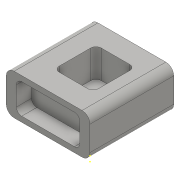
# Autodesk Inventor part: PassengerSection
Saved by Autodesk Inventor 2016 (Build 200138000, 138)
## iProperties
Created: 2016-01-08
Part Number: PassengerSection
Material: Generic
Document SubType Name: Modeling
Designer: 301278
Density: 1 g/cm^3
Appearance: Default
Author: 301278
Autodesk Inventor part; units mm, degrees
ref_plane "YZ Plane" through (0, 0, 0) normal (1, 0, 0) x (0, 1, 0)
ref_plane "XZ Plane" through (0, 0, 0) normal (0, 1, 0) x (-1, 0, 0)
ref_plane "XY Plane" through (0, 0, 0) normal (0, 0, 1) x (1, 0, 0)
sketch "Sketch1" plane through (0, 0, 0) normal (0, 0, 1) x (1, 0, 0)
  point P0 (0, 0)
sketch "Sketch2" plane through (0, 0, 0) normal (0, 0, 1) x (1, 0, 0)
  line L0 (7.62, 0) -> (72.898, 0)
  line L1 (80.518, 7.62) -> (80.518, 31.242)
  line L2 (72.898, 38.862) -> (7.62, 38.862)
  line L3 (0, 31.242) -> (0, 7.62)
  arc A0 (7.62, 38.862) -> (0, 31.242) centre (7.62, 31.242) ccw
  arc A1 (80.518, 31.242) -> (72.898, 38.862) centre (72.898, 31.242) ccw
  arc A2 (72.898, 0) -> (80.518, 7.62) centre (72.898, 7.62) ccw
  arc A3 (0, 7.62) -> (7.62, 0) centre (7.62, 7.62) ccw
  point P0 (0, 0)
  point P1 (80.518, 38.862)
  point P2 (80.518, 0)
  point P3 (0, 38.862)
  dimension "d0" = 80.518
  dimension "d1" = 38.862
  dimension "d2" = 7.62
  dimension "d3" = 7.62
  constraints: 8 end point, 8 point on circle, 8 point on line, 8 tangent, 4 centre point, 2 equal radius, 2 parallel, 1 horizontal, 1 perpendicular
  measures "d0" distance of point (0, 38.862) point (80.518, 38.862)
  measures "d1" distance of point (80.518, 38.862) point (80.518, 0)
  measures "d2" radius of A0
  measures "d3" radius of A1
extrude "Extrusion1" add sketch "Sketch2" along normal blind 80.518
sketch "Sketch3" plane through (0, 0, 80.518) normal (0, 0, 1) x (1, 0, 0)
  line L0 (13.716, 32.004) -> (66.802, 32.004)
  line L1 (71.882, 26.924) -> (71.882, 10.16)
  line L2 (66.802, 5.08) -> (13.716, 5.08)
  line L3 (8.636, 10.16) -> (8.636, 26.924)
  arc A0 (13.716, 32.004) -> (8.636, 26.924) centre (13.716, 26.924) ccw
  arc A1 (71.882, 26.924) -> (66.802, 32.004) centre (66.802, 26.924) ccw
  arc A2 (66.802, 5.08) -> (71.882, 10.16) centre (66.802, 10.16) ccw
  arc A3 (8.636, 10.16) -> (13.716, 5.08) centre (13.716, 10.16) ccw
  line L4 (72.898, 38.862) -> (7.62, 38.862) projected
  line L5 (0, 31.242) -> (0, 7.62) projected
  line L6 (80.518, 7.62) -> (80.518, 31.242) projected
  line L7 (72.898, 0) -> (7.62, 0) projected
  point P0 (0, 0)
  dimension "d6" = 5.08
  dimension "d7" = 5.08
  dimension "d8" = 6.858
  dimension "d9" = 8.636
  dimension "d10" = 8.636
  dimension "d11" = 5.08
  constraints: 8 end point, 8 point on circle, 8 tangent, 4 centre point, 2 equal radius, 2 parallel, 1 horizontal, 1 perpendicular
  measures "d6" radius of A0
  measures "d7" radius of A1
  measures "d8" distance between parallel lines of L4 L0
  measures "d9" distance between parallel lines of L5 L3
  measures "d10" distance between parallel lines of L6 L1
  measures "d11" distance from line of L7 L2.start
extrude "Extrusion2" cut sketch "Sketch3" against normal blind 14.478
sketch "Sketch4" plane through (0, 0, 0) normal (0, 0, -1) x (-1, 0, 0)
  line L0 (-65.659, 33.782) -> (-14.859, 33.782)
  line L1 (-9.779, 28.702) -> (-9.779, 10.16)
  line L2 (-14.859, 5.08) -> (-65.659, 5.08)
  line L3 (-70.739, 10.16) -> (-70.739, 28.702)
  arc A0 (-65.659, 33.782) -> (-70.739, 28.702) centre (-65.659, 28.702) ccw
  arc A1 (-70.739, 10.16) -> (-65.659, 5.08) centre (-65.659, 10.16) ccw
  arc A2 (-14.859, 5.08) -> (-9.779, 10.16) centre (-14.859, 10.16) ccw
  arc A3 (-9.779, 28.702) -> (-14.859, 33.782) centre (-14.859, 28.702) ccw
  line L4 (-7.62, 38.862) -> (-72.898, 38.862) projected
  line L5 (-72.898, 0) -> (-7.62, 0) projected
  line L6 (0, 7.62) -> (0, 31.242) projected
  line L7 (-80.518, 31.242) -> (-80.518, 7.62) projected
  point P0 (0, 0)
  dimension "d14" = 5.08
  dimension "d15" = 5.08
  dimension "d16" = 5.08
  dimension "d17" = 9.779
  dimension "d18" = 9.779
  constraints: 8 end point, 8 point on circle, 8 tangent, 4 centre point, 3 equal radius, 2 parallel, 1 horizontal, 1 perpendicular
  measures "d14" radius of A0
  measures "d15" distance between parallel lines of L4 L0
  measures "d16" distance between parallel lines of L5 L2
  measures "d17" distance between parallel lines of L6 L1
  measures "d18" distance between parallel lines of L7 L3
extrude "Extrusion3" cut sketch "Sketch4" against normal blind 14.478
sketch "Sketch5" plane through (14.859, 5.08, 0) normal (0, 1, 0) x (1, 0, 0)
  point P0 (-14.859, 0)
sketch "Sketch6" plane through (7.62, 38.862, 0) normal (0, 1, 0) x (1, 0, 0)
  line L0 (42.8172, -61.214) -> (15.357, -61.214)
  line L1 (10.277, -56.134) -> (10.277, -25.908)
  line L2 (15.357, -20.828) -> (42.8172, -20.828)
  line L3 (47.8972, -25.908) -> (47.8972, -56.134)
  arc A0 (42.8172, -61.214) -> (47.8972, -56.134) centre (42.8172, -56.134) ccw
  arc A1 (10.277, -56.134) -> (15.357, -61.214) centre (15.357, -56.134) ccw
  arc A2 (15.357, -20.828) -> (10.277, -25.908) centre (15.357, -25.908) ccw
  arc A3 (47.8972, -25.908) -> (42.8172, -20.828) centre (42.8172, -25.908) ccw
  line L4 (58.039, 0) -> (7.239, 0) projected
  point P0 (-7.62, 0)
  dimension "d21" = 5.08
  dimension "d22" = 40.386
  dimension "d23" = 20.828
  constraints: 8 end point, 8 point on circle, 8 tangent, 4 centre point, 3 equal radius, 2 parallel, 1 horizontal, 1 perpendicular
  measures "d21" radius of A0
  measures "d22" distance between parallel lines of L0 L2
  measures "d23" distance between parallel lines of L4 L2
extrude "Extrusion4" cut sketch "Sketch6" against normal blind 27.178
body "Solid1"
